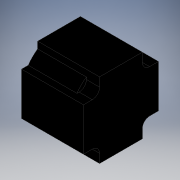
# Autodesk Inventor part: AKM2G-51DNCA_H
Saved by Autodesk Inventor 2019 (Build 230136000, 136)
## iProperties
Created: 2024-01-27
Part Number: AKM2G-51DNCA_H
Material: Generic
Catalog Web Link: www.cadenas.de
Description: AKM2G Size 5 - Housing-AKM2G Series
Vendor: KOLLMORGEN
Document SubType Name: Modeling
Designer: psAdmin
Manufacturer: KOLLMORGEN
Mass: 1032.02 g
Surface Area: 621.434 cm^2
Volume: 1032.02 cm^3
Density: 1 g/cm^3
Appearance: PSOLRGB-0-0-0
Category: PARTsolutions
Company: KOLLMORGEN
Title: AKM2G-51DNCA_H
Author: Cadenas PARTsolutions
Comments: AKM2G Series
PSOL_IDENT_0: {$CADENAS_DATA/23d-libs/kollmorgen/akm2g/parts/akm2g5_housing.prj},195 {VTYP=3D},{NB=AKM2G-51DNCA_H}
PSOL_IDENT_1: ,{LINA=AKM2G-51DNCA_H},{NN=AKM2G Size 5 - Housing},{DATE=28.07.2023 05:36:25},{GEOMDATE=28.07.2023 0
PSOL_IDENT_2: 5:25:00},{VERSION=},{LINEID=10},{WBVAR=L,BR,CON,FD},{WBNUMERIC=}  {NB=AKM2G-51DNCA_H},{LINA=AKM2G-51
PSOL_IDENT_3: DNCA_H},{KT=DUMMY},{PN=AKM2G-51DNCA},{FS=Size 5},{L=1},{MO=Metric IEC},{BR=N},{LX=94},{A=20},{CON=D}
PSOL_IDENT_4: ,{FD=CA},{FDALG='CA','Sfd3 smart feedback','GF','Multi-turn hiperface dsl','LD','Multi-turn inductiv
PSOL_IDENT_5: e endat 2.2'}
NB: AKM2G-51DNCA_H
NN: AKM2G Size 5 - Housing
NT: AKM2G Series
NBSYN: $PN._H
LINA: AKM2G-51DNCA_H
CATALOG: Kollmorgen
FS: Size 5
L: 1 Stack
MO: Metric IEC
BR: No brake
CON: Single right angle M23
FD: Sfd3 smart feedback
SUPPLIER: KOLLMORGEN
ARTICLENO: AKM2G-51DNCA_H
BOMINFO: AKM2G-51DNCA_H
CREATOR: CADENAS GmbH
Autodesk Inventor part; units mm, degrees
ref_plane "YZ Plane" through (0, 0, 0) normal (1, 0, 0) x (0, 1, 0)
ref_plane "XZ Plane" through (0, 0, 0) normal (0, 1, 0) x (-1, 0, 0)
ref_plane "XY Plane" through (0, 0, 0) normal (0, 0, 1) x (1, 0, 0)
sketch "Sketch_1" plane through (0, 0, 0) normal (1, 0, 0) x (0, 1, 0)
  line L0 (-32.5, 57) -> (-32.5, 43.5)
  arc A0 (-43.5, 32.5) -> (-32.5, 43.5) centre (-43.5, 43.5) ccw
  line L1 (-43.5, 32.5) -> (-57, 32.5)
  line L2 (-57, 32.5) -> (-57, -32.5)
  line L3 (-57, -32.5) -> (-43.5, -32.5)
  arc A1 (-32.5, -43.5) -> (-43.5, -32.5) centre (-43.5, -43.5) ccw
  line L4 (-32.5, -43.5) -> (-32.5, -57)
  line L5 (-32.5, -57) -> (32.5, -57)
  line L6 (32.5, -57) -> (32.5, -43.5)
  arc A2 (43.5, -32.5) -> (32.5, -43.5) centre (43.5, -43.5) ccw
  line L7 (43.5, -32.5) -> (57, -32.5)
  line L8 (57, -32.5) -> (57, 32.5)
  line L9 (57, 32.5) -> (43.5, 32.5)
  arc A3 (32.5, 43.5) -> (43.5, 32.5) centre (43.5, 43.5) ccw
  line L10 (32.5, 43.5) -> (32.5, 57)
  line L11 (32.5, 57) -> (-32.5, 57)
  constraints: 24 end point, 8 point on circle, 4 centre point
extrude "Extrusion1" add sketch "Sketch_1" along normal blind 94
sketch "Sketch_2" plane through (0, 0, 0) normal (1, 0, 0) x (0, 1, 0)
  circle A0 centre (0, 0) radius 57
  constraints: 1 centre point
extrude "Extrusion2" add sketch "Sketch_2" along normal blind 74
ref_plane "H1_XY" through (0, 0, 0) normal (1, 0, 0) x (0, 0, -1)
ref_plane "H1_YZ" through (0, 0, 0) normal (0, 0, -1) x (0, 1, 0)
ref_plane "H1_ZX" through (0, 0, 0) normal (0, 1, 0) x (1, 0, 0)
ref_plane "H2_XY" through (94, 0, 0) normal (-1, 0, 0) x (0, 0, -1)
ref_plane "H2_YZ" through (94, 0, 0) normal (0, 0, -1) x (0, -1, 0)
ref_plane "H2_ZX" through (94, 0, 0) normal (0, -1, 0) x (-1, 0, 0)
body "Solid1"
